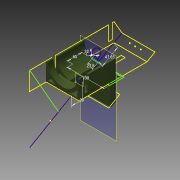
# Autodesk Inventor part: 知能ロボコン発射台改２.2
Saved by Autodesk Inventor 2013 (Build 170138000, 138)
## iProperties
Created: 2014-05-17
Part Number: 知能ロボコン発射台改２.2
Material: ABS プラスチック
Document SubType Name: Modeling
Designer: horumo136
Density: 1.06 g/cm^3
Mass: 430.971 g
Surface Area: 1189.26 cm^2
Volume: 406.576 cm^3
Author: horumo136
Autodesk Inventor part; units mm, degrees
ref_plane "YZ Plane" through (0, 0, 0) normal (1, 0, 0) x (0, 1, 0)
ref_plane "XZ Plane" through (0, 0, 0) normal (0, 1, 0) x (-1, 0, 0)
ref_plane "XY Plane" through (0, 0, 0) normal (0, 0, 1) x (1, 0, 0)
sketch "スケッチ1" plane through (0, 0, 0) normal (0, 1, 0) x (-1, 0, 0)
  line L0 (0, 0) -> (-90, 0)
  line L1 (-90, 0) -> (-90, 50)
  line L2 (0, 50) -> (0, 0)
  line L3 (0, 0) -> (-5, 0)
  line L4 (-5, 0) -> (-5, 50)
  line L5 (-5, 0) -> (-90, 0)
  line L6 (-90, 0) -> (-85, 0)
  line L7 (-85, 0) -> (-85, 50)
  arc A0 (-85, 50) -> (-5, 50) centre (-45, 50) ccw
  line L8 (0, 0) -> (0, 10)
  line L9 (0, 10) -> (-90, 10)
  circle A1 centre (-45, 50) radius 45
  line L10 (-90, 5) -> (0, 5)
  line L11 (-90, 50) -> (-85, 50)
  line L12 (-5, 50) -> (0, 50)
  line L13 (0, 0) -> (-90, 0)
  line L14 (-90, 0) -> (-90, 5)
  line L15 (-90, 5) -> (0, 5)
  line L16 (0, 5) -> (0, 0)
  dimension "d0" = 90
  dimension "d1" = 50
  dimension "d2" = 5
  dimension "d3" = 85
  dimension "d4" = 5
  dimension "d5" = 80
  dimension "d6" = 10
  dimension "d7" = 90
  constraints: 34 end point, 7 perpendicular, 5 parallel, 5 point on line, 2 centre point, 2 horizontal, 2 point on circle, 1 coincident, 1 collinear, 1 midpoint
  measures "d0" distance of L1.end L2.start
  measures "d1" distance of L0.end L1.end
  measures "d2" distance of L0.start L3.end
  measures "d3" distance of L3.end L0.end
  measures "d4" distance of L0.end L6.end
  measures "d5" diameter of A0
  measures "d6" distance of L0.start L8.end
  measures "d7" diameter of A1
extrude "押し出し1" add sketch "スケッチ1" along normal blind 230 contours L0 L4 L10 L2 | L0 L7 L10 L4 | L10 L4 L9 L2 | L0 L1 L10 L7 | L10 A1 L9 L4 | L9 L4 A1 L2 | L10 L1 L9 L7 | L7 L9 A1 L10 | L9 A1 L4 | A1 L9 | A1 L4 L12 | L9 L1 A1 L7 | L7 A1 L9 | A1 L9 A0 L4 | A1 L7 A0 L9 | L11 L7 A1
sketch "スケッチ2" plane through (0, 0, 0) normal (0, -1, 0) x (1, 0, 0)
  line L0 (0, 0) -> (0, 50) projected
  line L1 (90, 0) -> (0, 0) projected
  line L2 (90, 50) -> (90, 0) projected
  line L3 (85, 50) -> (90, 50) projected
  arc A0 (5, 50) -> (85, 50) centre (45, 50) ccw projected
  line L4 (0, 50) -> (5, 50) projected
  arc A1 (5, 23.467) -> (85, 23.467) centre (45, 50) ccw
  line L5 (0, 5) -> (90, 5)
  line L6 (5, 23.467) -> (5, 5)
  line L7 (85, 23.467) -> (85, 5)
  dimension "d29" = 48
  constraints: 8 end point, 4 point on line, 3 perpendicular, 2 point on circle, 2 tangent, 1 centre point, 1 coincident
  measures "d29" radius of A1
extrude "押し出し2" cut sketch "スケッチ2" against normal blind 225 contours L6 A1 L5 | L5 A1 L7
sketch "スケッチ3" plane through (0, 230, 0) normal (0, 1, 0) x (1, 0, 0)
  arc A0 (85, -50) -> (5, -50) centre (45, -50) ccw projected
  line L0 (90, -50) -> (90, 0) projected
  line L1 (0, -50) -> (5, -50) projected
  arc A1 (85, -50) -> (5, -50) centre (45, -50) ccw
  line L2 (5, -50) -> (85, -50)
  constraints: 3 end point, 2 point on circle, 1 centre point, 1 coincident, 1 perpendicular
extrude "押し出し3" add sketch "スケッチ3" against normal blind 5
sketch "スケッチ4" plane through (90, 0, 50) normal (1, 0, 0) x (0, 0, -1)
  line L0 (0, 0) -> (50, 0) projected
  line L1 (0, 0) -> (0, 230) projected
  line L2 (25, 0) -> (25, 60)
  line L3 (25, 60) -> (25, 70)
  line L4 (25, 70) -> (25, 210)
  line L5 (25, 210) -> (25, 220)
  line L6 (0, 60) -> (40, 60)
  line L7 (40, 60) -> (40, 70)
  line L8 (40, 70) -> (0, 70)
  line L9 (0, 70) -> (0, 60)
  line L10 (0, 215) -> (40, 215)
  line L11 (40, 215) -> (40, 225)
  line L12 (40, 225) -> (0, 225)
  line L13 (0, 225) -> (0, 215)
  dimension "d16" = 60
  dimension "d17" = 10
  dimension "d18" = 140
  dimension "d19" = 10
  dimension "d20" = 40
  dimension "d103" = 10
  dimension "d104" = 60
  constraints: 24 end point, 5 parallel, 3 collinear, 2 horizontal, 2 perpendicular, 2 point on line, 1 midpoint
  measures "d16" distance of L2.start L2.end
  measures "d17" distance of L2.end L3.end
  measures "d18" distance of L3.end L4.end
  measures "d19" distance of L4.end L5.end
  measures "d20" distance of L8.end L7.end
  measures "d103" distance between parallel lines of L6 L8
  measures "d104" distance between parallel lines of L0 L6
extrude "押し出し4" cut sketch "スケッチ4" against normal blind 90 contours L1 L8 L3 L6 | L3 L8 L7 L6 | L1 L12 L11 L10
sketch "スケッチ6" plane through (90, 0, 50) normal (1, 0, 0) x (0, 0, -1)
  line L0 (0, 230) -> (50, 230) projected
  line L1 (50, 230) -> (37.5, 251.6506)
  line L2 (50, 230) -> (110, 230) construction
  line L3 (0, 230) -> (37.5, 251.6506)
  line L4 (0, 230) -> (43.3013, 230) construction
  dimension "d32" = 120
  dimension "d33" = 30
  constraints: 8 end point, 2 horizontal, 1 equal length
  measures "d32" angle of L2 L1
  measures "d33" angle of L4 L3
extrude "押し出し6" add sketch "スケッチ6" against normal blind 90
sketch "スケッチ9" plane through (0, 0, 0) normal (-1, 0, 0) x (0, 0, 1)
  line L0 (10, 225) -> (50, 225) projected
  line L1 (50, 225) -> (50, 230) projected
  line L2 (50, 230) -> (12.5, 251.6506) projected
  line L3 (12.5, 251.6506) -> (0, 230) projected
  line L4 (0, 0) -> (0, 230) projected
  line L5 (0, 0) -> (50, 0) projected
  line L6 (50, 0) -> (50, 60) projected
  line L7 (50, 60) -> (10, 60) projected
  line L8 (10, 60) -> (10, 70) projected
  line L9 (10, 70) -> (50, 70) projected
  line L10 (50, 70) -> (50, 215) projected
  line L11 (50, 215) -> (10, 215) projected
  line L12 (10, 215) -> (10, 225) projected
  line L13 (12.5, 251.6506) -> (0, 230)
  line L14 (0, 230) -> (-132.7906, 0)
  line L15 (0, 145) -> (-49.0748, 145)
  line L16 (0, 115) -> (-66.3953, 115)
  dimension "d45" = 30
  constraints: 8 end point, 2 collinear, 2 midpoint, 2 point on line, 1 perpendicular
  measures "d45" distance between parallel lines of L15 L16
sketch "スケッチ10" plane through (0, 0, 0) normal (-1, 0, 0) x (0, 0, 1)
  line L0 (10, 225) -> (50, 225) projected
  line L1 (50, 225) -> (50, 230) projected
  line L2 (50, 230) -> (12.5, 251.6506) projected
  line L3 (12.5, 251.6506) -> (0, 230) projected
  line L4 (0, 0) -> (0, 230) projected
  line L5 (0, 0) -> (50, 0) projected
  line L6 (50, 0) -> (50, 60) projected
  line L7 (50, 60) -> (10, 60) projected
  line L8 (10, 60) -> (10, 70) projected
  line L9 (10, 70) -> (50, 70) projected
  line L10 (50, 70) -> (50, 215) projected
  line L11 (50, 215) -> (10, 215) projected
  line L12 (10, 215) -> (10, 225) projected
  line L13 (12.5, 251.6506) -> (-87.5, 78.4456)
  line L14 (-87.5, 78.4456) -> (50, 0)
  constraints: 4 end point, 1 collinear
sketch "スケッチ11" plane through (90, 230, 0) normal (0, 0.5, -0.8660254) x (-1, 0, 0)
  line L0 (0, 25) -> (90, 25) projected
  line L1 (45, 25) -> (45, 15)
  line L2 (45, 15) -> (60, 15)
  line L3 (60, 15) -> (30, 15)
  point P0 (90, -199.1858)
  dimension "d49" = 10
  dimension "d50" = 15
  dimension "d51" = 30
  constraints: 6 end point, 4 coincident, 2 perpendicular, 1 collinear, 1 midpoint
  measures "d49" distance of L1.start L1.end
  measures "d50" distance of L1.end L2.end
  measures "d51" distance of L2.end L3.end
hole "穴1" at (45, 242.9904, 7.5) at (30, 242.9904, 7.5) at (60, 242.9904, 7.5) direction (0, -0.5, 0.8660254) diameter 2.5 depth 8 tip angle 118
sketch "スケッチ18" plane through (90, 60, 10) normal (0, 0, 1) x (1, 0, 0)
  line L0 (0, 10) -> (-5, 10) projected
  line L1 (0, 10) -> (-90, 10)
  line L2 (-90, 10) -> (-90, 150)
  line L3 (-90, 150) -> (0, 150)
  line L4 (0, 150) -> (0, 10)
  line L5 (-45, 150) -> (-45, 10)
  line L6 (-53.1517, 150) -> (-27.646, 150)
  line L7 (-27.646, 150) -> (-27.646, 10)
  line L8 (-27.646, 10) -> (-53.1517, 10)
  line L9 (-53.1517, 10) -> (-53.1517, 150)
  line L10 (-45, 10) -> (-39.75, 10)
  line L11 (-45, 150) -> (-50.25, 150)
  line L12 (-50.25, 150) -> (-39.75, 150)
  line L13 (-39.75, 150) -> (-39.75, 10)
  line L14 (-39.75, 10) -> (-50.25, 10)
  line L15 (-50.25, 10) -> (-50.25, 150)
  point P0 (-90, -60)
  dimension "d76" = 140
  dimension "d77" = 5.25
  dimension "d78" = 5.25
  constraints: 30 end point, 6 parallel, 4 point on line, 3 perpendicular, 2 horizontal, 2 midpoint, 1 collinear
  measures "d76" distance of L1.end L2.end
  measures "d77" distance of L5.end L10.end
  measures "d78" distance of L5.start L11.end
extrude "押し出し12" cut sketch "スケッチ18" against normal blind 10 and the other way blind 5 contours L1 L5 L3 L13 | L1 L15 L3 L5
sketch "スケッチ19" plane through (0, 0, 0) normal (-1, 0, 0) x (0, 0, 1)
  line L0 (10, 225) -> (50, 225) projected
  line L1 (50, 225) -> (50, 230) projected
  line L2 (50, 230) -> (12.5, 251.6506) projected
  line L3 (12.5, 251.6506) -> (0, 230) projected
  line L4 (0, 0) -> (0, 230) projected
  line L5 (0, 0) -> (50, 0) projected
  line L6 (50, 0) -> (50, 60) projected
  line L7 (50, 60) -> (10, 60) projected
  line L8 (10, 60) -> (10, 70) projected
  line L9 (10, 70) -> (50, 70) projected
  line L10 (50, 70) -> (50, 215) projected
  line L11 (50, 215) -> (10, 215) projected
  line L12 (10, 215) -> (10, 225) projected
  line L13 (0, 230) -> (-23.825, 188.7339)
  line L14 (-23.825, 188.7339) -> (-3.4734, 176.9839)
  circle A0 centre (-3.4734, 176.9839) radius 16
  circle A1 centre (-3.4734, 176.9839) radius 3
  dimension "d83" = 47.65
  dimension "d84" = 23.5
  dimension "d85" = 32
  dimension "d86" = 6
  constraints: 4 end point, 3 coincident, 2 centre point, 1 collinear, 1 perpendicular
  measures "d83" distance of L3.end L13.end
  measures "d84" distance of L13.end L14.end
  measures "d85" diameter of A0
  measures "d86" diameter of A1
sketch "スケッチ20" plane through (90, 230, 0) normal (0, 0.5, -0.8660254) x (-1, 0, 0)
  circle A0 centre (60, 15) radius 1.25 projected
  circle A1 centre (45, 15) radius 1.25 projected
  circle A2 centre (30, 15) radius 1.25 projected
  line L0 (0, 0) -> (0, 25) projected
  line L1 (0, 0) -> (90, 0) projected
  line L2 (90, 25) -> (90, 0) projected
  line L3 (0, 25) -> (90, 25) projected
  point P0 (90, -199.1858)
ref_plane "作業平面5" through (90, 45, 50) normal (0, 1, 0) x (1, 0, 0)
sketch "スケッチ21" plane through (90, 45, 50) normal (0, 1, 0) x (1, 0, 0)
  line L0 (0, 0) -> (-101.8599, 0)
  line L1 (-101.8599, 0) -> (-101.8599, 60.1995)
  line L2 (-101.8599, 60.1995) -> (0, 60.1995)
  line L3 (0, 60.1995) -> (0, 0)
  point P0 (-90, 50)
  constraints: 8 end point, 2 parallel, 1 horizontal, 1 perpendicular
extrude "押し出し13" cut sketch "スケッチ21" against normal blind 50
ref_plane "作業平面6" through (85, 142.5, 23.467) normal (0, 1, 0) x (-1, 0, 0)
sketch "スケッチ22" plane through (0, 70, 50) normal (-1, 0, 0) x (0, 0, 1)
  line L0 (-37.5, 181.6506) -> (-50, 160) projected
  line L1 (-50, -25) -> (-50, 160) projected
  line L2 (-98.8395, 70.6051) -> (-50, 70.6051)
  line L3 (-107.0544, 55.6051) -> (-50, 55.6051)
  line L4 (-89.7339, 85.6051) -> (-50, 85.6051)
  line L5 (-89.7339, 85.6051) -> (-107.0544, 55.6051)
  line L6 (-50, 55.6051) -> (-50, 85.6051)
  point P0 (-50, -70)
  dimension "d90" = 30
  dimension "d92" = 15
  constraints: 10 end point, 3 perpendicular, 3 point on line, 1 collinear, 1 parallel
  measures "d90" distance between parallel lines of L3 L4
  measures "d92" distance between parallel lines of L2 L4
extrude "押し出し14" add sketch "スケッチ22" against normal blind 90
sketch "スケッチ23" plane through (0, 125.6051, -57.0544) normal (0, -1, 0) x (1, 0, 0)
  line L0 (0, 0) -> (90, 0) projected
  line L1 (39.75, 57.0544) -> (50.25, 57.0544) projected
  line L2 (45, 57.0544) -> (45, 0)
  line L3 (37.5, 57.0544) -> (52.5, 57.0544)
  line L4 (52.5, 57.0544) -> (52.5, 0)
  line L5 (52.5, 0) -> (37.5, 0)
  line L6 (37.5, 0) -> (37.5, 57.0544)
  line L7 (37.5, 57.0544) -> (52.5, 0) construction
  line L8 (52.5, 57.0544) -> (37.5, 0) construction
  line L9 (37.5, 57.0544) -> (52.5, 57.0544)
  line L10 (52.5, 57.0544) -> (52.5, 37.0544)
  line L11 (52.5, 37.0544) -> (37.5, 37.0544)
  line L12 (37.5, 37.0544) -> (37.5, 57.0544)
  point P0 (45, 28.5272)
  dimension "d95" = 15
  dimension "d96" = 20
  constraints: 22 end point, 5 midpoint, 4 parallel, 2 horizontal, 2 perpendicular, 2 point on line
  measures "d95" distance of L4.end L5.end
  measures "d96" distance of L9.end L10.end
extrude "押し出し15" cut sketch "スケッチ23" against normal blind 90 contours L6 L3 L1 L2 L11 | L2 L1 L3 L4 L11
sketch "スケッチ24" plane through (90, 230, 0) normal (0, 0, -1) x (-1, 0, 0)
  line L0 (50.25, -20) -> (50.25, -160) projected
  line L1 (50.25, -160) -> (39.75, -160) projected
  line L2 (39.75, -160) -> (39.75, -20) projected
  line L3 (39.75, -20) -> (50.25, -20) projected
  line L4 (52.5, -104.3949) -> (52.5, -74.3949) projected
  line L5 (52.5, -74.3949) -> (90, -74.3949) projected
  line L6 (90, -74.3949) -> (90, 0) projected
  line L7 (0, 0) -> (90, 0) projected
  line L8 (0, -74.3949) -> (0, 0) projected
  line L9 (0, -74.3949) -> (37.5, -74.3949) projected
  line L10 (37.5, -104.3949) -> (37.5, -74.3949) projected
  line L11 (37.5, -104.3949) -> (0, -104.3949) projected
  line L12 (0, -185) -> (0, -104.3949) projected
  line L13 (0, -185) -> (90, -185) projected
  line L14 (90, -185) -> (90, -104.3949) projected
  line L15 (90, -104.3949) -> (52.5, -104.3949) projected
  line L16 (0, -104.3949) -> (90, -104.3949)
  line L17 (90, -104.3949) -> (90, -74.3949)
  line L18 (90, -74.3949) -> (0, -74.3949)
  line L19 (0, -74.3949) -> (0, -104.3949)
  line L20 (-5, -66.8949) -> (95, -66.8949)
  line L21 (95, -66.8949) -> (95, -106.8949)
  line L22 (95, -106.8949) -> (-5, -106.8949)
  line L23 (-5, -106.8949) -> (-5, -66.8949)
  line L24 (-5, -66.8949) -> (95, -106.8949) construction
  line L25 (95, -66.8949) -> (-5, -106.8949) construction
  line L26 (0, -69.3949) -> (90, -69.3949)
  line L27 (90, -69.3949) -> (90, -104.3949)
  line L28 (90, -104.3949) -> (0, -104.3949)
  line L29 (0, -104.3949) -> (0, -69.3949)
  line L30 (0, -69.3949) -> (90, -104.3949) construction
  line L31 (90, -69.3949) -> (0, -104.3949) construction
  point P0 (90, -230)
  point P1 (45, -86.8949)
  dimension "d99" = 100
  dimension "d100" = 40
  constraints: 32 end point, 6 parallel, 4 midpoint, 3 horizontal, 3 perpendicular
  measures "d99" distance of L21.end L22.end
  measures "d100" distance of L20.end L21.end
sketch "スケッチ25" plane through (90, 155.6051, -39.7339) normal (0, 0.5, -0.8660254) x (-1, 0, 0)
  line L0 (90, 0) -> (90, -34.641) projected
  line L1 (90, 0) -> (0, 0) projected
  line L2 (0, -34.641) -> (0, 0) projected
  line L3 (90, -34.641) -> (0, -34.641) projected
  point P0 (90, -114.891)
sketch "スケッチ26" plane through (85, 142.5, 23.467) normal (0, 1, 0) x (-1, 0, 0)
  line L0 (125.1914, -92.9646) -> (-58.6843, -92.9646)
  line L1 (-58.6843, -92.9646) -> (-58.6843, 63.112)
  line L2 (-58.6843, 63.112) -> (125.1914, 63.112)
  line L3 (125.1914, 63.112) -> (125.1914, -92.9646)
  point P0 (85, -23.467)
  constraints: 8 end point, 2 parallel, 1 horizontal, 1 perpendicular
extrude "押し出し16" cut sketch "スケッチ26" along normal blind 110
sketch "スケッチ27" plane through (0, 60, 10) normal (-1, 0, 0) x (0, 0, 1)
  line L0 (40, 82.5) -> (-57.3001, 82.5) projected
  line L1 (-57.3001, 82.5) -> (-67.0544, 65.6051) projected
  line L2 (40, 10) -> (40, 82.5) projected
  line L3 (-10, 82.5) -> (-10, 87.5)
  line L4 (-10, 87.5) -> (-54.4134, 87.5)
  line L5 (-57.3001, 82.5) -> (-54.4134, 87.5)
  line L6 (-44.3714, 87.5) -> (-44.3714, 82.5)
  point P0 (-10, -60)
  dimension "d105" = 5
  constraints: 8 end point, 3 point on line, 2 perpendicular, 1 collinear, 1 parallel
  measures "d105" distance of L3.start L3.end
sketch "スケッチ28" plane through (85, 142.5, 23.467) normal (0, 1, 0) x (1, 0, 0)
  line L0 (-85, 70.7671) -> (5, 70.7671) projected
  line L1 (-85, -26.533) -> (-85, 70.7671) projected
  line L2 (-80, -26.533) -> (-85, -26.533) projected
  arc A0 (-45.25, 13.121) -> (-80, -26.533) centre (-40, -26.533) ccw projected
  line L3 (-45.25, 23.467) -> (-45.25, 13.121) projected
  line L4 (-47.5, 23.467) -> (-45.25, 23.467) projected
  line L5 (-47.5, 43.467) -> (-47.5, 23.467) projected
  line L6 (-32.5, 43.467) -> (-47.5, 43.467) projected
  line L7 (-32.5, 23.467) -> (-32.5, 43.467) projected
  line L8 (-34.75, 23.467) -> (-32.5, 23.467) projected
  line L9 (-34.75, 13.121) -> (-34.75, 23.467) projected
  arc A1 (0, -26.533) -> (-34.75, 13.121) centre (-40, -26.533) ccw projected
  line L10 (5, -26.533) -> (0, -26.533) projected
  line L11 (5, 70.7671) -> (5, -26.533) projected
  line L12 (0, 18.467) -> (-23.2967, 18.467) projected
  line L13 (0, 0) -> (0, 18.467) projected
  arc A2 (0, 0) -> (-23.2967, 18.467) centre (-40, -26.533) ccw projected
  line L14 (-56.7033, 18.467) -> (-80, 18.467) projected
  arc A3 (-56.7033, 18.467) -> (-80, 0) centre (-40, -26.533) ccw projected
  line L15 (-80, 18.467) -> (-80, 0) projected
  line L16 (-85, 70.7671) -> (5, 70.7671)
  line L17 (5, 70.7671) -> (5, 60.7671)
  line L18 (5, 60.7671) -> (-85, 60.7671)
  line L19 (-85, 60.7671) -> (-85, 70.7671)
  point P0 (-85, 23.467)
  dimension "d106" = 10
  constraints: 8 end point, 2 parallel, 1 horizontal, 1 perpendicular, 1 point on line
  measures "d106" distance of L16.end L17.end
extrude "押し出し17" add sketch "スケッチ28" along normal blind 5 contours L18 L11 L10 A1 L9 L8 L7 L6 L5 L4 L3 A0 L2 L1
extrude "押し出し18" add sketch "スケッチ27" against normal blind 90 contours L0 L5 L4 L6
sketch "スケッチ29" plane through (90, 60, 10) normal (1, 0, 0) x (0, 0, -1)
  line L0 (10, 65.6051) -> (67.0544, 65.6051)
  line L1 (67.0544, 65.6051) -> (67.0544, 70.6051)
  line L2 (67.0544, 70.6051) -> (10, 70.6051)
  line L3 (10, 70.6051) -> (10, 65.6051)
  point P0 (10, -60)
  dimension "d111" = 5
  constraints: 8 end point, 2 parallel, 1 horizontal, 1 perpendicular
  measures "d111" distance of L1.end L0.end
extrude "押し出し19" cut sketch "スケッチ29" against normal blind 90
sketch "スケッチ30" plane through (90, 60, 10) normal (1, 0, 0) x (0, 0, -1)
  line L0 (64.1677, 70.6051) -> (54.4134, 87.5) projected
  line L1 (10, -15) -> (10, 70.6051) projected
  line L2 (54.4134, 87.5) -> (56.5784, 88.75)
  line L3 (56.5784, 88.75) -> (67.6119, 69.6395)
  line L4 (67.6119, 69.6395) -> (65.4468, 68.3895)
  line L5 (65.4468, 68.3895) -> (54.4134, 87.5)
  line L6 (54.4134, 87.5) -> (57.3001, 87.5)
  line L7 (64.1677, 70.6051) -> (67.0544, 70.6051)
  point P0 (10, -60)
  dimension "d114" = 2.5
  constraints: 12 end point, 3 parallel, 3 perpendicular, 2 point on line
  measures "d114" distance of L0.end L2.end
extrude "押し出し20" add sketch "スケッチ30" against normal blind 90 contours L0 L6 L3 L7
sketch "スケッチ31" plane through (90, 60, 10) normal (1, 0, 0) x (0, 0, -1)
  line L0 (-40, 87.5) -> (76.2018, 87.5)
  line L1 (76.2018, 87.5) -> (76.2018, 85)
  line L2 (76.2018, 85) -> (-40, 85)
  line L3 (-40, 85) -> (-40, 87.5)
  point P0 (10, -60)
  dimension "d117" = 2.5
  constraints: 8 end point, 2 parallel, 1 horizontal, 1 perpendicular
  measures "d117" distance of L0.end L1.end
extrude "押し出し21" cut sketch "スケッチ31" against normal blind 90
sketch "スケッチ32" plane through (90, 130.6051, -57.0544) normal (0, 0.5, -0.8660254) x (-1, 0, 0)
  line L0 (90, 16.6218) -> (0, 16.6218) projected
  line L1 (0, 0) -> (0, 16.6218) projected
  line L2 (0, 0) -> (90, 0) projected
  line L3 (90, 16.6218) -> (90, 0) projected
  point P0 (90, -84.5801)
extrude "押し出し22" add sketch "スケッチ32" along normal blind 3
